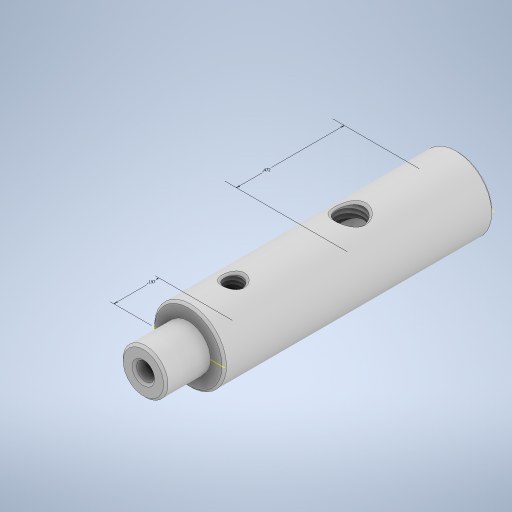
# Autodesk Inventor part: BT802_goteln20_21_Zeichenmaschine_Welle_2zu5
Saved by Autodesk Inventor 2023 (Build 270158000, 158)
## iProperties
Created: 2023-01-08
Part Number: BT802_goteln20_21_Zeichenmaschine_Welle_2zu5
Material: Generisch
Document SubType Name: Modeling
Designer: eligo
Density: 1 g/cm^3
Appearance: Vorgabe
Author: eligo
Autodesk Inventor part; units mm, degrees
ref_plane "YZ Plane" through (0, 0, 0) normal (1, 0, 0) x (0, 1, 0)
ref_plane "XZ Plane" through (0, 0, 0) normal (0, 1, 0) x (-1, 0, 0)
ref_plane "XY Plane" through (0, 0, 0) normal (0, 0, 1) x (1, 0, 0)
sketch "Skizze1" plane through (0, 0, 0) normal (1, 0, 0) x (0, 1, 0)
  line L0 (0, 20) -> (0, -20)
  line L1 (0, 5) -> (2.5, 5)
  line L2 (2.5, 5) -> (2.5, 0)
  line L3 (2.5, 0) -> (0, 0) construction
  line L4 (2.5, 0) -> (4, 0)
  line L5 (4, 0) -> (4, -30)
  line L6 (4, -30) -> (0, -30)
  line L7 (2.5, -8) -> (2.5, -30)
  line L8 (1, 5) -> (1, -8)
  line L9 (1, -8) -> (2.5, -8)
  dimension "d0" = 40
  dimension "d1" = 5
  dimension "d2" = 5
  dimension "d4" = 8
  dimension "d5" = 30
  dimension "d8" = 22
  dimension "d9" = 5
  dimension "d10" = 2
  constraints: 20 end point, 5 perpendicular, 4 point on line, 2 horizontal, 2 parallel, 1 coincident, 1 midpoint, 1 vertical
  measures "d0" distance of L0.start L0.end
  measures "d1" distance of L1.end L2.end
  measures "d2" diameter of L2 L0
  measures "d4" diameter of L5 L0
  measures "d5" distance of L4.end L5.end
  measures "d8" distance of L7.start L7.end
  measures "d9" diameter of L7 L0
  measures "d10" diameter of L8 L0
revolve "Umdrehung1" add sketch "Skizze1" angle 360 about axis through (0, 0, 20) along (0, 0, -1)
sketch "Skizze2" plane through (0, 0, 0) normal (0, 1, 0) x (-1, 0, 0)
  line L0 (-4, -30) -> (4, -30) projected
  line L1 (-4, 0) -> (4, 0) projected
  point P0 (0, 0)
  point P1 (0, -5)
  point P2 (0, -18)
  dimension "d12" = 12
  dimension "d13" = 5
  measures "d12" distance from line of point (0, -18) L0
  measures "d13" distance from line of point (0, -5) L1
hole "Bohrung1" at (0, 0, -5) direction (0, 1, 0) diameter 2 end through all
hole "Bohrung2" at (0, 0, -18) direction (0, 1, 0) diameter 3 end through all
thread "Gewinde1" size "M3x0.5" class "6H" standard "ISO Metric profile" full length
thread "Gewinde2" size "M2x0.4" class "6H" standard "ISO Metric profile" full length
chamfer "Fase1" distance 0.25 angle 45 2 edges at (1.5, 3.7081, -18.0006) (-1.5, 3.7081, -17.9994)
chamfer "Fase2" distance 0.25 angle 45 2 edges at (1, 3.873, -4.9999) (-1, 3.873, -5.0001)
chamfer "Fase3" distance 0.25 angle 45 1 edges at (0, -1, 5)
chamfer "Fase4" distance 0.25 angle 45 1 edges at (0, -2.5, -30)
chamfer "Fase5" distance 0.25 angle 45 1 edges at (0, -2.5, 5)
chamfer "Fase6" distance 0.25 angle 45 1 edges at (0, -4, 0)
chamfer "Fase7" distance 0.25 angle 45 1 edges at (0, -4, -30)
